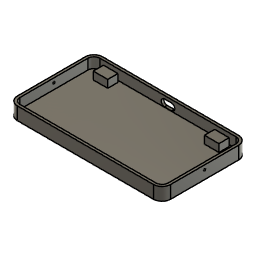
Case (15mm Thickness) (Autodesk Fusion 360 design; units mm, degrees)
Autodesk Fusion 360 part; units mm, degrees
sketch "Walls" plane through (0, 0, 0) normal (0, 1, 0) x (1, 0, 0)
  line L0 (-80, 50) -> (80, 50)
  line L1 (90, 40) -> (90, -40)
  line L2 (80, -50) -> (-80, -50)
  line L3 (-90, -40) -> (-90, 40)
  line L4 (-90, 50) -> (90, -50) construction
  line L5 (90, 50) -> (-90, -50) construction
  arc A0 (-90, -40) -> (-80, -50) centre (-80, -40) ccw
  arc A1 (80, -50) -> (90, -40) centre (80, -40) ccw
  arc A2 (90, 40) -> (80, 50) centre (80, 40) ccw
  arc A3 (-80, 50) -> (-90, 40) centre (-80, 40) ccw
  arc A4 (87, 40) -> (80, 47) centre (80, 40) ccw
  line L6 (-80, 47) -> (80, 47)
  arc A5 (-80, 47) -> (-87, 40) centre (-80, 40) ccw
  line L7 (-87, -40) -> (-87, 40)
  arc A6 (-87, -40) -> (-80, -47) centre (-80, -40) ccw
  line L8 (80, -47) -> (-80, -47)
  arc A7 (80, -47) -> (87, -40) centre (80, -40) ccw
  line L9 (87, 40) -> (87, -40)
  dimension "d1" = 180
  dimension "d2" = 100
  dimension "d3" = 10
  dimension "d4" = 3
  constraint horizontal L0
  constraint perpendicular L0 L1
  constraint parallel L0 L2
  constraint parallel L1 L3
  constraint coincident L4 origin
  constraint coincident L5 origin
  constraint coincident L5.end L3
  constraint coincident L5.end L2
  constraint tangent L3 A0
  constraint tangent L2 A0
  constraint coincident L4.end L2
  constraint coincident L4.end L1
  constraint tangent L2 A1
  constraint tangent L1 A1
  constraint equal A0 A1
  constraint coincident L5.start L1
  constraint coincident L5.start L0
  constraint tangent L1 A2
  constraint tangent L0 A2
  constraint equal A0 A2
  constraint coincident L4.start L0
  constraint coincident L4.start L3
  constraint tangent L0 A3
  constraint tangent L3 A3
  constraint equal A0 A3
  measures "d1" distance of L4.end L5.end
  measures "d2" distance of L5.start L4.end
  measures "d3" radius of A0
extrude "Floor Extrusion" add sketch "Walls" along normal blind 3 contours L0 L1 L2 L3 A0 A1 A2 A3 | A4 L6 A5 L7 A6 L8 A7 L9
extrude "Walls Extrusion" add sketch "Walls" along normal blind 15
sketch "Port" plane through (0, 0, -50) normal (0, 0, -1) x (-1, 0, 0)
  line L0 (-80, 0) -> (80, 0)
  line L1 (80, 0) -> (80, 15)
  line L2 (80, 15) -> (-80, 15)
  line L3 (-80, 15) -> (-80, 0)
  line L4 (4, 11.5) -> (-4, 11.5)
  arc A0 (-4, 11.5) -> (-4, 3.5) centre (-4, 7.5) ccw
  line L5 (-4, 3.5) -> (4, 3.5)
  arc A1 (4, 3.5) -> (4, 11.5) centre (4, 7.5) ccw
  line L6 (4, 7.5) -> (-4, 7.5) construction
  line L7 (80, 0) -> (-80, 0)
  dimension "d11" = 8
  dimension "d12" = 8
  dimension "d25" = 4
  dimension "d42" = 7.5
  constraint tangent L4 A0
  constraint tangent A0 L5
  constraint parallel L4 L5
  constraint tangent L5 A1
  constraint tangent L4 A1
  constraint horizontal L6
  measures "d11" distance of A1.centre A0.centre
  measures "d12" diameter of A0
  measures "d25" horizontal distance of origin A0.end
  measures "d42" distance of L6 L7
extrude "Port Extrusion" cut sketch "Port" against normal blind 3 contours L4 A0 L5 A1
sketch "Tab Holes" plane through (0, 0, 0) normal (1, 0, 0) x (0, 0, -1)
  circle A0 centre (0, 10) radius 1.25
  line L0 (-40, 15) -> (40, 15)
  dimension "d26" = 2.5
  dimension "d27" = 5
  measures "d26" diameter of A0
  measures "d27" distance of A0.centre L0
extrude "Tab Holes Extrusion" cut sketch "Tab Holes" along normal through all and the other way through all
sketch "Encoder Blocks" plane through (0, 3, 0) normal (0, 1, 0) x (-1, 0, 0)
  line L0 (87, -40) -> (87, 40)
  arc A0 (87, 40) -> (80, 47) centre (80, 40) ccw
  line L1 (80, 47) -> (-80, 47)
  arc A1 (-80, 47) -> (-87, 40) centre (-80, 40) ccw
  line L2 (-87, 40) -> (-87, -40)
  arc A2 (-87, -40) -> (-80, -47) centre (-80, -40) ccw
  line L3 (-80, -47) -> (80, -47)
  arc A3 (80, -47) -> (87, -40) centre (80, -40) ccw
  line L4 (73.8, -45) -> (56.8, -45)
  line L5 (56.8, -45) -> (56.8, -33)
  line L6 (56.8, -33) -> (73.8, -33)
  line L7 (73.8, -33) -> (73.8, -45)
  line L8 (73.8, -45) -> (56.8, -33) construction
  line L9 (56.8, -45) -> (73.8, -33) construction
  line L10 (80, -50) -> (-80, -50)
  line L11 (90, 40) -> (90, -40)
  line L12 (-56.8, -45) -> (-73.8, -33) construction
  line L13 (-56.8, -33) -> (-56.8, -45)
  line L14 (-56.8, -45) -> (-73.8, -45)
  line L15 (-73.8, -45) -> (-56.8, -33) construction
  line L16 (-73.8, -33) -> (-56.8, -33)
  line L17 (-73.8, -45) -> (-73.8, -33)
  line L18 (80, -47) -> (-80, -47)
  line L19 (-90, -40) -> (-90, 40)
  point P0 (65.3, -39)
  point P1 (-65.3, -39)
  dimension "d29" = 17
  dimension "d30" = 12
  dimension "d31" = 5
  dimension "d32" = 16.2
  dimension "d35" = 17
  dimension "d36" = 12
  dimension "d38" = 5
  dimension "d39" = 16.2
  constraint horizontal L4
  constraint perpendicular L4 L5
  constraint parallel L4 L6
  constraint parallel L5 L7
  constraint coincident L8 P0
  constraint coincident L9 P0
  constraint horizontal L14
  constraint perpendicular L14 L17
  constraint parallel L14 L16
  constraint parallel L13 L17
  constraint coincident P1 L12
  constraint coincident P1 L15
  measures "d29" distance of L5.end L6.end
  measures "d30" distance of L4.end L5.end
  measures "d31" distance of L4 L10
  measures "d32" distance of L7 L11
  measures "d35" distance of L12.end L13.start
  measures "d36" distance of L14.end L12.end
  measures "d38" distance of L10 L14
  measures "d39" distance of L17 L19
extrude "Left Encoder Block Extrusion" add sketch "Encoder Blocks" along normal blind 9 contours L4 L5 L6 L7
extrude "Right Encoder Block Extrusion" add sketch "Encoder Blocks" along normal blind 9 contours L13 L14 L16 L17
equation "d25 = ( 8 / 2 ) * 1 mm"
equation "d27 = ( 10 / 2 ) * 1 mm"
equation "d33 = 15 mm - 3 mm - 3 mm"
equation "d40 = 15 mm - 3 mm - 3 mm"
equation "d42 = ( 15 / 2 ) * 1 mm"
named bodies: "Body"
